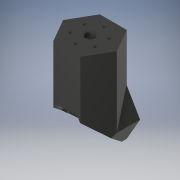
# Autodesk Inventor part: TARM01
Saved by Autodesk Inventor 2017 (Build 210142000, 142)
## iProperties
Created: 2018-10-11
Part Number: TARM01
Material: ABS Plastic
Document SubType Name: Modeling
Designer: Zach
Density: 1.06 g/cm^3
Appearance: Smooth - Black
Author: Zach
Autodesk Inventor part; units mm, degrees
ref_plane "YZ Plane" through (0, 0, 0) normal (1, 0, 0) x (0, 1, 0)
ref_plane "XZ Plane" through (0, 0, 0) normal (0, 1, 0) x (-1, 0, 0)
ref_plane "XY Plane" through (0, 0, 0) normal (0, 0, 1) x (1, 0, 0)
sketch "Sketch9" plane through (0, 0, 0) normal (0, 0, 1) x (1, 0, 0)
  line L0 (56, 0) -> (28, -48.4974)
  line L1 (28, -48.4974) -> (-28, -48.4974)
  line L2 (-28, -48.4974) -> (-56, 0)
  line L3 (-56, 0) -> (-28, 48.4974)
  line L4 (-28, 48.4974) -> (28, 48.4974)
  line L5 (28, 48.4974) -> (56, 0)
  circle A0 centre (25.9808, 15) radius 2.5
  circle A1 centre (0, 0) radius 10
  circle A2 centre (0, 30) radius 2.5
  circle A3 centre (-25.9808, 15) radius 2.5
  circle A4 centre (-25.9808, -15) radius 2.5
  circle A5 centre (0, -30) radius 2.5
  circle A6 centre (25.9808, -15) radius 2.5
  dimension "d52" = 112
  dimension "d53" = 5
  dimension "d54" = 30
  dimension "d55" = 20
  dimension "d58" = 360
  constraints: 12 end point, 7 centre point, 2 coincident, 1 horizontal alignment, 1 vertical alignment, 26 other
  measures "d52" distance of L0.start L2.end
  measures "d53" diameter of A0
  measures "d54" distance of A0.centre point (0, 0)
  measures "d55" diameter of A1
extrude "Extrusion7" add sketch "Sketch9" along normal blind 96.995
sketch "Sketch10" plane through (0, 0, 96.995) normal (0, 0, 1) x (1, 0, 0)
  line L0 (28, -48.4974) -> (56, 0) projected
  line L1 (56, 0) -> (56, 48.4974)
  line L2 (28, 48.4974) -> (-28, 48.4974) projected
  line L3 (56, 48.4974) -> (28, 48.4974)
  line L4 (-28, 48.4974) -> (-56, 0) projected
  line L5 (-56, 0) -> (-56, 48.4974)
  line L6 (-56, 48.4974) -> (-28, 48.4974)
  line L7 (56, 0) -> (28, 48.4974) projected
  point P0 (0, 0)
  constraints: 8 end point, 2 perpendicular, 2 vertical
extrude "Extrusion8" add sketch "Sketch10" against normal blind 96.995
sketch "Sketch11" plane through (-56, 48.4974, 0) normal (0, 1, 0) x (1, 0, 0)
  line L0 (112.0001, -48.4975) -> (84, -96.995)
  line L1 (84, -96.995) -> (28, -96.995)
  line L2 (28, -96.995) -> (-0.0001, -48.4975)
  line L3 (-0.0001, -48.4975) -> (28, 0)
  line L4 (28, 0) -> (84, 0)
  line L5 (84, 0) -> (112.0001, -48.4975)
  line L6 (0, 0) -> (112, 0) projected
  line L7 (0, -96.995) -> (0, 0) projected
  line L8 (112, -96.995) -> (0, -96.995) projected
  line L9 (112, -96.995) -> (112, 0) projected
  line L10 (0, -96.995) -> (0, 0) projected
  line L11 (-0.0001, -48.4975) -> (0, -96.995)
  line L12 (0, -96.995) -> (0, -96.995)
  line L13 (112, -96.995) -> (0, -96.995) projected
  line L14 (28, -96.995) -> (0, -96.995)
  line L15 (0, 0) -> (112, 0) projected
  line L16 (-0.0001, -48.4975) -> (0, 0)
  line L17 (0, 0) -> (28, 0)
  line L18 (84, 0) -> (112, 0)
  line L19 (112, 0) -> (112.0001, -48.4975)
  line L20 (112.0001, -48.4975) -> (112, -96.995)
  line L21 (112, -96.995) -> (84, -96.995)
  point P0 (56, -48.4975)
  point P1 (56, 0)
  constraints: 30 end point, 3 horizontal alignment, 2 collinear, 2 midpoint, 1 horizontal, 13 other
extrude "Extrusion9" cut sketch "Sketch11" against normal through all contours L9 L8 L0 | L5 L6 L9 | L8 L7 L2 | L3 L7 L6
sketch "Sketch12" plane through (-28, 48.4974, 96.995) normal (0, 1, 0) x (1, 0, 0)
  circle A0 centre (28, 48.4973) radius 10
  line L0 (0, 96.995) -> (56.0001, 96.995) projected
  circle A1 centre (28, 78.4973) radius 2.5
  circle A2 centre (2.0193, 63.4973) radius 2.5
  circle A3 centre (2.0193, 33.4973) radius 2.5
  circle A4 centre (28, 18.4973) radius 2.5
  circle A5 centre (53.9808, 33.4973) radius 2.5
  circle A6 centre (53.9808, 63.4973) radius 2.5
  point P0 (28, 96.995)
  point P1 (28, 96.995)
  point P2 (84, 48.4973)
  dimension "d66" = 20
  dimension "d67" = 5
  dimension "d68" = 30
  dimension "d71" = 360
  constraints: 7 centre point, 2 vertical alignment, 1 horizontal alignment, 1 midpoint, 13 other
  measures "d66" diameter of A0
  measures "d67" diameter of A1
  measures "d68" distance of A0.centre A1.centre
extrude "Extrusion10" cut sketch "Sketch12" against normal through all
chamfer "Chamfer2" distance 48.4973 angle 45 1 edges at (0, -48.4974, 96.995)
sketch "Sketch14" plane through (-28, 48.4974, 96.995) normal (0, 1, 0) x (1, 0, 0)
  circle A0 centre (53.9808, 63.4973) radius 2.5 projected
  circle A1 centre (28, 18.4973) radius 2.5 projected
  circle A2 centre (2.0193, 63.4973) radius 2.5 projected
  circle A3 centre (28, 78.4973) radius 2.5 projected
  circle A4 centre (2.0193, 33.4973) radius 2.5 projected
  circle A5 centre (53.9808, 33.4973) radius 2.5 projected
  circle A6 centre (28, 48.4973) radius 10 projected
  line L0 (0, 96.995) -> (-28, 48.4977) projected
  line L1 (-28, 48.4973) -> (-28, 48.4977) projected
  line L2 (-28, 48.4973) -> (0, 0) projected
  line L3 (56.0001, 0) -> (0, 0) projected
  line L4 (56.0001, 0) -> (84, 48.4973) projected
  line L5 (84, 48.4973) -> (84, 48.4977) projected
  line L6 (84, 48.4977) -> (56.0001, 96.995) projected
  line L7 (0, 96.995) -> (56.0001, 96.995) projected
  point P0 (28, 96.995)
extrude "Extrusion12" add sketch "Sketch14" along normal blind 100
sketch "Sketch15" plane through (0, 0, 0) normal (0, 0, -1) x (-1, 0, 0)
  line L0 (56, 0) -> (28, -48.4974)
  line L1 (28, -48.4974) -> (-28, -48.4974)
  line L2 (-28, -48.4974) -> (-56, 0)
  line L3 (-56, 0) -> (-28, 48.4974)
  line L4 (-28, 48.4974) -> (28, 48.4974)
  line L5 (28, 48.4974) -> (56, 0)
  circle A0 centre (0, 0) radius 10 projected
  circle A1 centre (0, 30) radius 2.5 projected
  circle A2 centre (0, 30) radius 2.5
  circle A3 centre (-25.9808, 15) radius 2.5
  circle A4 centre (-25.9808, -15) radius 2.5
  circle A5 centre (0, -30) radius 2.5
  circle A6 centre (25.9808, -15) radius 2.5
  circle A7 centre (25.9808, 15) radius 2.5
  dimension "d87" = 360
  constraints: 12 end point, 6 centre point, 2 coincident, 1 concentric, 26 other
extrude "Extrusion13" add sketch "Sketch15" against normal blind 48.4973
sketch "Sketch16" plane through (0, 0, 96.995) normal (0, 0, 1) x (1, 0, 0)
  arc A0 (-10, 0) -> (10, 0) centre (0, 0) ccw projected
  line L0 (-28, -48.4974) -> (-56, 0) projected
  line L1 (-56, 0) -> (-28, 48.4974)
  line L2 (-28, 48.4974) -> (28, 48.4974)
  line L3 (28, 48.4974) -> (56, 0)
  line L4 (56, 0) -> (28, -48.4974)
  line L5 (28, -48.4974) -> (-28, -48.4974)
  line L6 (-28, -48.4974) -> (-56, 0)
  line L7 (-22.2265, 38.4974) -> (-44.453, 0)
  line L8 (-44.453, 0) -> (-22.2265, -38.4974)
  line L9 (-22.2265, -38.4974) -> (22.2265, -38.4974)
  line L10 (22.2265, -38.4974) -> (44.453, 0)
  line L11 (44.453, 0) -> (22.2265, 38.4974)
  line L12 (22.2265, 38.4974) -> (-22.2265, 38.4974)
  line L13 (-44.453, 0) -> (-56, 0)
  line L14 (56, 0) -> (42, -24.2487) projected
  line L15 (56, 0) -> (44.453, 0)
  point P0 (0, 0)
  dimension "d91" = 10
  constraints: 28 end point, 1 coincident, 1 collinear, 1 horizontal, 18 other
  measures "d91" distance between parallel lines of L1 L7
extrude "Extrusion14" cut sketch "Sketch16" against normal blind 86.9947 contours L0 L13 L8 L9 L10 L15 L4 L5 | L7 L12 L11 L10 L9 L8
sketch "Sketch17" plane through (0, 0, 10.0003) normal (0, 0, 1) x (1, 0, 0)
  line L0 (-28, 28.4973) -> (-22.2265, 38.4974) projected
  line L1 (-28, -48.4974) -> (-56, 0) projected
  line L2 (-28, 28.4973) -> (-28, -48.4974)
  line L3 (28, 28.4973) -> (44.453, 0) projected
  line L4 (28, 28.4973) -> (28, -48.4974)
  line L5 (56, 0) -> (28, -48.4974) projected
  line L6 (44.453, 0) -> (56, 0) projected
  line L7 (-44.453, 0) -> (-28, 28.4973) projected
  line L8 (-56, 0) -> (-44.453, 0) projected
  point P0 (0, 0)
  constraints: 4 end point
extrude "Extrusion15" add sketch "Sketch17" along normal blind 86.9947
sketch "Sketch18" plane through (-28, -48.4974, 10.0003) normal (1, 0.0000006, 0) x (0, 0, -1)
  line L0 (0, 76.9948) -> (0, 64.9714) projected
  line L1 (-52.0234, 76.9948) -> (0, 76.9948) projected
  line L2 (-52.0234, 76.9948) -> (-54.9713, 76.9948) projected
  line L3 (-86.9947, 76.9948) -> (-54.9713, 76.9948) projected
  line L4 (-86.9947, 0) -> (-86.9947, 76.9948) projected
  line L5 (0, 0) -> (-86.9947, 0) projected
  line L6 (0, 32.0234) -> (0, 0) projected
  line L7 (0, 34.9714) -> (0, 32.0234) projected
  line L8 (0, 62.0235) -> (0, 34.9714) projected
  line L9 (0, 64.9714) -> (0, 62.0235) projected
  line L10 (-58.4973, 48.4974) -> (-86.9947, 76.9948) projected
  line L11 (0, 0) -> (-86.9947, 76.9948)
  line L12 (-86.9947, 48.4974) -> (-86.9947, 0) projected
  line L13 (-86.9947, 0) -> (0, 0)
  line L14 (0, 0) -> (0, -25)
  line L15 (0, -25) -> (-86.9947, -25)
  line L16 (-86.9947, -25) -> (-86.9947, 0)
  point P0 (10.0003, 48.4974)
  dimension "d98" = 25
  constraints: 10 end point, 2 parallel, 1 horizontal, 1 perpendicular, 1 vertical alignment
  measures "d98" distance of L15.end L4.start
extrude "Extrusion16" cut sketch "Sketch18" along normal through all both and the other way through all contours L11 L5 L4 | L14 L15 L16 L5
sketch "Sketch20" plane through (56, 0, 64.7964) normal (0, 1, 0) x (1, 0, 0)
  line L0 (-9.4101, 0) -> (0, 0) projected
  line L1 (0, 16.2988) -> (0, 0) projected
  line L2 (-9.4101, 0) -> (0, 16.2988) projected
  line L3 (-112, -0.0001) -> (-102.5899, -0.0001) projected
  line L4 (-112, 16.2988) -> (-102.5899, -0.0001) projected
  line L5 (-112, 16.2988) -> (-112, -0.0001) projected
  point P0 (-56, 64.7964)
extrude "Extrusion17" cut sketch "Sketch20" against normal through all
sketch "Sketch21" plane through (-22.2265, 38.4974, 96.995) normal (0, -1, 0) x (1, 0, 0)
  circle A0 centre (22.2265, -48.4973) radius 10 projected
  circle A1 centre (48.2073, -33.4973) radius 2.5 projected
  circle A2 centre (-3.7543, -33.4973) radius 2.5 projected
  circle A3 centre (22.2265, -78.4973) radius 2.5 projected
  circle A4 centre (-3.7543, -63.4973) radius 2.5 projected
  circle A5 centre (22.2265, -18.4973) radius 2.5 projected
  circle A6 centre (48.2073, -63.4973) radius 2.5 projected
  line L0 (-5.7735, -96.995) -> (-33.7735, -48.4977) projected
  line L1 (-33.7735, -48.4977) -> (-33.7735, -48.4973) projected
  line L2 (-33.7735, -48.4973) -> (-5.7735, 0) projected
  line L3 (-5.7735, 0) -> (50.2265, 0) projected
  line L4 (50.2265, 0) -> (78.2265, -48.4973) projected
  line L5 (78.2265, -48.4973) -> (78.2265, -48.4977) projected
  line L6 (78.2265, -48.4977) -> (50.2265, -96.995) projected
  line L7 (50.2265, -96.995) -> (-5.7735, -96.995) projected
  line L8 (44.453, -10) -> (0, -10)
  line L9 (0, -10) -> (-22.2266, -48.4975)
  line L10 (-22.2266, -48.4975) -> (0, -86.995)
  line L11 (0, -86.995) -> (44.453, -86.995)
  line L12 (44.453, -86.995) -> (66.6796, -48.4975)
  line L13 (66.6796, -48.4975) -> (44.453, -10)
  point P0 (22.2265, -96.995)
  dimension "d101" = 10
  constraints: 12 end point, 5 other
  measures "d101" distance between parallel lines of L3 L8
extrude "Extrusion18" cut sketch "Sketch21" against normal blind 100 and the other way blind 100 contours A0 | A1 | A2 | A3 | A4 | A5 | A6 | L13 L12 L11 L10 L9 L8
sketch "Sketch22" plane through (-22.2265, -48.4974, 10) normal (0, 0, 1) x (1, 0, 0)
  line L0 (50.2266, 0) -> (50.2265, 0) projected
  line L1 (50.2265, 0) -> (-5.7735, 0)
  line L2 (-5.7735, 0) -> (-33.7735, 48.4974)
  line L3 (-33.7735, 48.4974) -> (-5.7735, 96.9948)
  line L4 (-5.7735, 96.9948) -> (50.2265, 96.9948)
  line L5 (50.2265, 96.9948) -> (78.2265, 48.4974)
  line L6 (78.2265, 48.4974) -> (50.2265, 0)
  line L7 (0, 10) -> (44.453, 10)
  line L8 (44.453, 10) -> (66.6795, 48.4974)
  line L9 (66.6795, 48.4974) -> (44.453, 86.9948)
  line L10 (44.453, 86.9948) -> (0, 86.9948)
  line L11 (0, 86.9948) -> (-22.2265, 48.4974)
  line L12 (-22.2265, 48.4974) -> (0, 10)
  point P0 (22.2265, 48.4974)
  point P1 (22.2265, 48.4974)
  dimension "d106" = 10
  constraints: 24 end point, 1 coincident, 18 other
  measures "d106" distance between parallel lines of L1 L7
extrude "Extrusion19" cut sketch "Sketch22" along normal through all contours L12 L11 L10 L9 L8 L7
sketch "Sketch24" plane through (-28, -48.4974, 10.0003) normal (0.0000004, -0.7488345, 0.662757) x (0.9339615, 0.2368522, 0.2676135)
  line L0 (10.7845, 61.8599) -> (10.7845, 74.2228) projected
  line L1 (10.7845, 74.2228) -> (41.5173, 108.5015) projected
  line L2 (41.5173, 108.5015) -> (0, 65.9865) projected
  line L3 (0, 0) -> (0, 65.9865) projected
  line L4 (4.7722, 12.4717) -> (0, 0) projected
  line L5 (4.7722, 12.4717) -> (3.0058, 53.8944) projected
  line L6 (3.0058, 53.8944) -> (10.7845, 61.8599) projected
  line L7 (93.8192, 42.4501) -> (85.5665, 33.2451) projected
  line L8 (85.5665, 33.2451) -> (86.0408, 22.1217) projected
  line L9 (86.0408, 22.1217) -> (57.0741, -7.5412) projected
  line L10 (52.3019, -20.0129) -> (57.0741, -7.5412) projected
  line L11 (52.3019, -20.0129) -> (52.3019, -20.0129) projected
  line L12 (96.3509, 29.1185) -> (52.3019, -20.0129) projected
  line L13 (96.3509, 29.1185) -> (93.8192, 88.4886) projected
  line L14 (93.8192, 88.4886) -> (93.8192, 88.4886) projected
  line L15 (93.8192, 42.4501) -> (93.8192, 88.4886) projected
  line L16 (41.5173, 108.5015) -> (0, 65.9865) projected
  line L17 (0, 65.9865) -> (10.7845, 61.8599)
  line L18 (85.5665, 33.2451) -> (89.4574, 31.051) projected
  line L19 (85.5665, 33.2451) -> (96.3509, 29.1185)
  circle A0 centre (5.3922, 63.9232) radius 2.5
  circle A1 centre (90.9587, 31.1818) radius 2.5
  point P0 (34.9614, 13.0189)
  dimension "d109" = 5
  dimension "d110" = 5
  constraints: 4 end point, 2 centre point, 2 midpoint, 1 collinear
  measures "d109" diameter of A0
  measures "d110" diameter of A1
extrude "Extrusion20" cut sketch "Sketch24" against normal blind 25 contours A0 L17 | L17 A0 | A1 L19 | A1 L19
body "Solid2"
